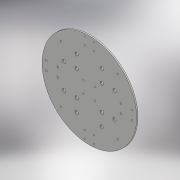
# Autodesk Inventor part: 底层板
Saved by Autodesk Inventor 2017 (Build 210142000, 142)
## iProperties
Part Number: 底层板
Material: 常规
Document SubType Name: Modeling
Designer: PANDA
Density: 1 g/cm^3
Appearance: 默认
Author: PANDA
Autodesk Inventor part; units mm, degrees
ref_plane "YZ Plane" through (0, 0, 0) normal (1, 0, 0) x (0, 1, 0)
ref_plane "XZ Plane" through (0, 0, 0) normal (0, 1, 0) x (-1, 0, 0)
ref_plane "XY Plane" through (0, 0, 0) normal (0, 0, 1) x (1, 0, 0)
sketch "草图1" plane through (0, 0, 0) normal (0, 1, 0) x (-1, 0, 0)
  circle A0 centre (0, 0) radius 150
  dimension "d0" = 300
  constraints: 1 centre point, 1 coincident
  measures "d0" diameter of A0
extrude "拉伸1" add sketch "草图1" along normal blind 4
sketch "草图2" plane through (0, 4, 0) normal (0, 1, 0) x (1, 0, 0)
  circle A0 centre (15, -140) radius 1.75
  circle A1 centre (-15, -140) radius 1.75
  circle A2 centre (15, 140) radius 1.75
  circle A3 centre (-15, 140) radius 1.75
  circle A4 centre (15, 116) radius 1.75
  circle A5 centre (-15, 116) radius 1.75
  circle A6 centre (-15, -116) radius 1.75
  circle A7 centre (15, -116) radius 1.75
  point P0 (0, 0)
  dimension "d3" = 3.5
  dimension "d4" = 3.5
  dimension "d5" = 3.5
  dimension "d6" = 3.5
  dimension "d7" = 3.5
  dimension "d8" = 3.5
  dimension "d9" = 3.5
  dimension "d10" = 3.5
  constraints: 8 centre point
  measures "d3" diameter of A0
  measures "d4" diameter of A1
  measures "d5" diameter of A2
  measures "d6" diameter of A3
  measures "d7" diameter of A4
  measures "d8" diameter of A5
  measures "d9" diameter of A6
  measures "d10" diameter of A7
hole "孔1" at (-15, 4, 140) at (-15, 4, 116) at (15, 4, 140) at (15, 4, 116) at (-15, 4, -116) at (-15, 4, -140) at (15, 4, -140) at (15, 4, -116) direction (0, -1, 0) diameter 3.5 end through all
sketch "草图3" plane through (0, 4, 0) normal (0, 1, 0) x (1, 0, 0)
  circle A0 centre (136, 14) radius 2.5
  circle A1 centre (136, -14) radius 2.5
  circle A2 centre (100, 14) radius 2.5
  circle A3 centre (100, -14) radius 2.5
  circle A4 centre (-100, -14) radius 2.5
  circle A5 centre (-100, 14) radius 2.5
  circle A6 centre (-136, -14) radius 2.5
  circle A7 centre (-136, 14) radius 2.5
  point P0 (0, 0)
  dimension "d18" = 5
  dimension "d19" = 5
  dimension "d20" = 5
  dimension "d21" = 5
  dimension "d22" = 5
  dimension "d23" = 5
  dimension "d24" = 5
  dimension "d25" = 5
  constraints: 8 centre point
  measures "d18" diameter of A0
  measures "d19" diameter of A1
  measures "d20" diameter of A2
  measures "d21" diameter of A3
  measures "d22" diameter of A4
  measures "d23" diameter of A5
  measures "d24" diameter of A6
  measures "d25" diameter of A7
hole "孔2" at (-136, 4, 14) at (-136, 4, -14) at (-100, 4, 14) at (-100, 4, -14) at (100, 4, 14) at (100, 4, -14) at (136, 4, 14) at (136, 4, -14) direction (0, -1, 0) diameter 5 end through all
sketch "草图4" plane through (0, 4, 0) normal (0, 1, 0) x (1, 0, 0)
  circle A0 centre (18.5, 18.5) radius 2
  circle A1 centre (18.5, -18.5) radius 2
  circle A2 centre (-18.5, 18.5) radius 2
  circle A3 centre (-18.5, -18.5) radius 2
  point P0 (0, 0)
  dimension "d33" = 4
  dimension "d34" = 4
  dimension "d35" = 4
  dimension "d36" = 4
  constraints: 4 centre point
  measures "d33" diameter of A0
  measures "d34" diameter of A1
  measures "d35" diameter of A2
  measures "d36" diameter of A3
hole "孔3" at (-18.5, 4, 18.5) at (-18.5, 4, -18.5) at (18.5, 4, -18.5) at (18.5, 4, 18.5) direction (0, -1, 0) diameter 4 end through all
sketch "草图5" plane through (0, 4, 0) normal (0, 1, 0) x (1, 0, 0)
  circle A0 centre (90, 90) radius 2.5
  circle A1 centre (-90, -90) radius 2.5
  circle A2 centre (90, -90) radius 2.5
  circle A3 centre (-90, 90) radius 2.5
  point P0 (0, 0)
  dimension "d44" = 5
  dimension "d45" = 5
  dimension "d46" = 5
  dimension "d47" = 5
  constraints: 4 centre point
  measures "d44" diameter of A0
  measures "d45" diameter of A1
  measures "d46" diameter of A2
  measures "d47" diameter of A3
hole "孔4" at (-90, 4, 90) at (-90, 4, -90) at (90, 4, -90) at (90, 4, 90) direction (0, -1, 0) diameter 5 end through all
sketch "草图6" plane through (0, 4, 0) normal (0, 1, 0) x (1, 0, 0)
  circle A0 centre (40, -40) radius 2.5
  circle A1 centre (40, 40) radius 2.5
  circle A2 centre (-40, 40) radius 2.5
  circle A3 centre (-40, -40) radius 2.5
  point P0 (0, 0)
  dimension "d55" = 5
  dimension "d56" = 5
  dimension "d57" = 5
  dimension "d58" = 5
  constraints: 4 centre point
  measures "d55" diameter of A0
  measures "d56" diameter of A1
  measures "d57" diameter of A2
  measures "d58" diameter of A3
hole "孔5" at (-40, 4, 40) at (-40, 4, -40) at (40, 4, -40) at (40, 4, 40) direction (0, -1, 0) diameter 10 end through all
sketch "草图7" plane through (0, 4, 0) normal (0, 1, 0) x (1, 0, 0)
  circle A0 centre (40, 80) radius 2.5
  circle A1 centre (80, 40) radius 2.5
  circle A2 centre (-40, -80) radius 2.5
  circle A3 centre (-80, -40) radius 2.5
  circle A4 centre (-40, 80) radius 2.5
  circle A5 centre (-80, 40) radius 2.5
  circle A6 centre (40, -80) radius 2.5
  circle A7 centre (80, -40) radius 2.5
  point P0 (0, 0)
  dimension "d66" = 5
  dimension "d67" = 5
  dimension "d68" = 5
  dimension "d69" = 5
  dimension "d70" = 5
  dimension "d71" = 5
  dimension "d72" = 5
  dimension "d73" = 5
  constraints: 8 centre point
  measures "d66" diameter of A0
  measures "d67" diameter of A1
  measures "d68" diameter of A2
  measures "d69" diameter of A3
  measures "d70" diameter of A4
  measures "d71" diameter of A5
  measures "d72" diameter of A6
  measures "d73" diameter of A7
hole "孔6" at (-80, 4, 40) at (-40, 4, 80) at (40, 4, 80) at (80, 4, 40) at (80, 4, -40) at (40, 4, -80) at (-40, 4, -80) at (-80, 4, -40) direction (0, -1, 0) diameter 10 end through all
